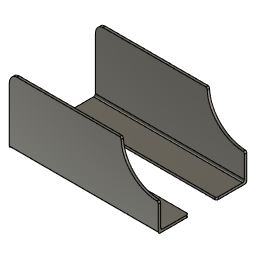
8in Rectangular Splitter End Plate (Autodesk Fusion 360 design; units mm, degrees)
Autodesk Fusion 360 part; units mm, degrees
note: some values were not read from the file. Set by a fixed rule: which sketch regions a step uses.
sketch "Sketch1" plane through (0, 0, 0) normal (0, 1, 0) x (1, 0, 0)
  line L0 (0, 0) -> (0, -88.9)
  line L1 (254, 0) -> (254, -38.1)
  line L2 (190.5, -88.9) -> (0, -88.9)
  line L3 (0, -88.9) -> (190.5, -88.9)
  ellipse E0 centre (254, -88.9) end of major axis (190.5, -88.9) minor radius 50.8 (254, -38.1) -> (190.5, -88.9) ccw
  line L4 (0, 0) -> (254, 0)
  dimension "d2" = 88.9
  dimension "d3" = 190.5
  constraint coincident L0.start L4.start
  constraint perpendicular L1 L4
  measures "d2" distance of L0.start L0.end
  measures "d3" distance of L0.end L2.start
extrude "Extrude3" add sketch "Sketch1" along normal blind 3.175 makes body 1
sketch "Sketch2" plane through (0, 3.175, 0) normal (0, 1, 0) x (-1, 0, 0)
  line L0 (0, 88.9) -> (-190.5, 88.9)
  ellipse E0 centre (-254, 88.9) end of major axis (-190.5, 88.9) minor radius 50.8 (-254, 38.1) -> (-190.5, 88.9) ccw
  line L1 (-254, 38.1) -> (-254, 0)
  line L2 (-254, 0) -> (0, 0)
  line L3 (0, 0) -> (0, 88.9)
  line L4 (-254, 0) -> (-254, 3.175)
  line L5 (-254, 3.175) -> (0, 3.175)
  line L6 (0, 0) -> (0, 3.175)
  line L7 (0, 0) -> (-254, 0)
  dimension "d11" = 3.175
  constraint coincident L1.end L2.start
  constraint perpendicular L2 L4
  constraint coincident L3 L5.end
  constraint perpendicular L3 L5
  constraint coincident L2.end L3.start
  measures "d11" distance of L1.end L4.end
extrude "Extrude4" add sketch "Sketch2" along normal blind 38.1 contours L1 L2 L3 L4 L5 L6 L7 bodies 1
fillet "Fillet1" radius 2.54 6 edges at (127, 3.175, 3.175) (127, 0, 0) (254, 1.5875, 38.1) (190.5, 1.5875, 88.9) (254, 41.275, 1.5875) (0, 41.275, 1.5875) on bodies 1
fillet "Fillet2" radius 12.7 1 edges at (0, 1.5875, 88.9) on bodies 1
mirror "Mirror1" about plane through (0, 41.275, 0) normal (0, 1, 0) of bodies 1 makes body 2
move_body "Move1" bodies 2 to x (1, 0, 0) y (0, 1, 0) z (0, 0, 1) at (0, 38.1, 0)
scale "Scale1" factors (0.8, 1, 1) about (0, 117.475, 5.715) bodies 1 2
